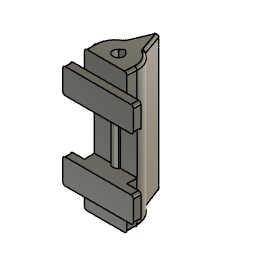
strumballz v18 (Autodesk Fusion 360 design; units mm, degrees)
Autodesk Fusion 360 part; units mm, degrees
note: some values were not read from the file. Chosen so that the rebuilt part matches the saved one: which sketch regions a step uses; which face or edge a step refers to; which pieces of a blend or face edit are solid.
sketch "Sketch1" plane through (0, 0, 0) normal (0, 0, 1) x (1, 0, 0)
  circle A0 centre (0, 0) radius 8.5
  line L0 (0, 8.5) -> (0, 18.5) construction
  line L1 (-8.400646, -4.05702) -> (8.400646, -4.05702)
  line L2 (8.400646, -4.05702) -> (8.497313, -0.213724)
  line L3 (-8.400646, -4.05702) -> (-8.497313, -0.213724)
  line L4 (0, 18.5) -> (-8.400646, -4.05702)
  line L5 (8.400646, -4.05702) -> (0, 18.5)
  dimension "d1" = 17
  dimension "d2" = 10
  constraint coincident A0.centre origin
  constraint coincident A0 L0.start
  constraint vertical L0
  constraint horizontal L1
  constraint tangent A0 L2
  constraint tangent A0 L3
  measures "d1" diameter of A0
  measures "d2" distance of L0.start L0.end
extrude "Extrude1" add sketch "Sketch1" along normal blind 55 contours A0 L5 | A0 L2 L5 | A0 L1 L5 | A0 L1 L4 L5 | A0 L4 L5 | A0 L4 | A0 L1 L4 | A0 L3 L4 picked at (5.724066, 3.776087) picked at (8.210444, -3.009315) picked at (7.842583, -3.934324) picked at (0.204704, 0.121249) picked at (0, 11.818524) picked at (-7.263613, 1.901443) picked at (-7.842583, -3.934324) picked at (-8.210444, -3.009315)
fillet "Fillet1" radius 1 1 edges at (0, 18.5, 27.5)
sketch "Sketch2" plane through (0, 0, 55) normal (0, 0, 1) x (-1, 0, 0)
  arc A0 (-0.937122, -15.983684) -> (0.937122, -15.983684) centre (0, -15.634682) ccw
  line L0 (0.937122, -15.983684) -> (4.121133, -7.434128)
  arc A1 (4.121133, -7.434128) -> (8.497313, 0.213724) centre (0, 0) ccw
  line L1 (8.497313, 0.213724) -> (8.400646, 4.05702)
  line L2 (8.400646, 4.05702) -> (-8.400646, 4.05702)
  line L3 (-8.400646, 4.05702) -> (-8.497313, 0.213724)
  arc A2 (-8.497313, 0.213724) -> (-4.121133, -7.434128) centre (0, 0) ccw
  line L4 (-4.121133, -7.434128) -> (-0.937122, -15.983684)
  line L5 (0, 4.05702) -> (0, -0.94298) construction
  circle A3 centre (0, -0.94298) radius 2.125
  line L6 (0, -3.801151) -> (-1.421105, -2.522881)
  line L7 (0, -3.801151) -> (1.421105, -2.522881)
  dimension "d7" = 5
  dimension "d8" = 4.25
  constraint perpendicular L2 L5
  constraint tangent A3 L6
  constraint tangent A3 L7
  measures "d8" diameter of A3
extrude "Extrude2" cut sketch "Sketch2" against normal up to surface (55 mm away) contours A3 | A3 L6 L7 picked at (0.385258, -0.460245) picked at (0.103405, -3.304782)
fillet "Fillet2" radius 0.5 2 edges at (-4.121133, 7.434128, 27.5) (4.121133, 7.434128, 27.5)
sketch "Sketch3" plane through (0, -4.05702, 0) normal (0, -1, 0) x (1, 0, 0)
  line L0 (-8.400646, 0) -> (8.400646, 0)
  line L1 (8.400646, 0) -> (8.400646, 55)
  line L2 (8.400646, 55) -> (-8.400646, 55)
  line L3 (-8.400646, 55) -> (-8.400646, 0)
  line L4 (0, 55) -> (0, 46.5) construction
  line L5 (0, 0) -> (0, 8.5) construction
  line L6 (14, 55.000001) -> (-14, 55.000001)
  line L7 (-14, 55.000001) -> (-14, 37.999999)
  line L8 (-14, 37.999999) -> (14, 37.999999)
  line L9 (14, 37.999999) -> (14, 55.000001)
  line L10 (14, 55.000001) -> (-14, 37.999999) construction
  line L11 (-14, 55.000001) -> (14, 37.999999) construction
  line L12 (14, 0) -> (-14, 0)
  line L13 (-14, 0) -> (-14, 17)
  line L14 (-14, 17) -> (14, 17)
  line L15 (14, 17) -> (14, 0)
  line L16 (14, 0) -> (-14, 17) construction
  line L17 (-14, 0) -> (14, 17) construction
  line L18 (2, 55.000001) -> (2, 48.000001) construction
  line L19 (14, 48.000001) -> (-14, 48.000001)
  line L20 (13, 0) -> (13, 7) construction
  line L21 (14, 7) -> (-14, 7)
  point P0 (0, 46.5)
  point P1 (0, 8.5)
  dimension "d14" = 8.5
  dimension "d15" = 8.5
  dimension "d36" = 7
  constraint midpoint L2 L4.start
  constraint perpendicular L2 L4
  constraint coincident L5.start origin
  constraint perpendicular L0 L5
  constraint horizontal L6
  constraint perpendicular L6 L7
  constraint parallel L6 L8
  constraint parallel L7 L9
  constraint coincident L10 P0
  constraint coincident L11 P0
  constraint coincident P0 L4.end
  constraint horizontal L12
  constraint perpendicular L12 L13
  constraint parallel L12 L14
  constraint parallel L13 L15
  constraint coincident L16 P1
  constraint coincident L17 P1
  constraint coincident P1 L5.end
  constraint perpendicular L7 L19
  constraint coincident L12 L20.start
  constraint coincident L15 L21.start
  constraint coincident L13 L21.end
  constraint perpendicular L13 L21
  measures "d14" distance of L4.start P0
  measures "d15" distance of L5.start P1
extrude "Extrude3" add sketch "Sketch3" along normal blind 3 contours L3 L13 L14 L21 | L1 L3 L14 L21 | L1 L14 L15 L21 | L3 L7 L8 L19 | L1 L3 L8 L19 | L1 L8 L9 L19 picked at (-10.267098, 10.333333) picked at (2.800215, 10.333333) picked at (10.267098, 13.666667) picked at (-10.267098, 44.666667) picked at (-2.800215, 41.333333) picked at (12.133549, 41.333333)
sketch "Sketch4" plane through (0, -4.05702, 0) normal (0, -1, 0) x (1, 0, 0)
  line L0 (-8.400646, 17) -> (8.400646, 17)
  line L1 (8.400646, 17) -> (8.400646, 37.999999)
  line L2 (8.400646, 37.999999) -> (-8.400646, 37.999999)
  line L3 (-8.400646, 37.999999) -> (-8.400646, 17)
  line L4 (-10, 38.000001) -> (10, 38.000001)
  line L5 (10, 38.000001) -> (10, 17)
  line L6 (10, 17) -> (-10, 17)
  line L7 (-10, 17) -> (-10, 38.000001)
  constraint horizontal L4
  constraint vertical L5
  constraint horizontal L6
  constraint vertical L7
extrude "Extrude4" cut sketch "Sketch4" against normal blind 4 contours L0 L1 L2 L3 L4 L6 | L3 L4 L6 L7 | L1 L4 L5 L6 picked at (2.800215, 24) picked at (-9.466882, 31) picked at (9.466882, 24)
draft "Draft1" angle -2 neutral plane through (0, -0.05702, 0) pull (0, -1, 0) 2 faces at (0.312374, 10.397575, 55) (0.312374, 10.397575, 0)
fillet "Fillet3" radius 1 4 edges at (14, -5.55702, 17) (14, -5.55702, 37.999999) (-14, -5.55702, 37.999999) (-14, -5.55702, 17)
fillet "Fillet4" radius 1 4 edges at (-14, -5.55702, 7) (14, -5.55702, 7) (-14, -5.55702, 48.000001) (14, -5.55702, 48.000001)
fillet "Fillet5" radius 1 11 edges at (8.44898, -2.135372, 55.072578) (-2.497399, 11.794102, 54.58615) (-4.143869, 7.456849, 54.73761) (-7.382537, 4.212854, 54.850893) (-8.498922, -0.135377, 55.002736) (-8.44898, -2.135372, 55.072578) (8.498922, -0.135377, 55.002736) (7.382537, 4.212854, 54.850893) (4.143869, 7.456849, 54.73761) (2.497399, 11.794102, 54.58615) (0, 16.634682, 54.417113)
fillet "Fillet6" radius 1 11 edges at (-2.497399, 11.794102, 0.41385) (-4.143869, 7.456849, 0.26239) (-7.382537, 4.212854, 0.149107) (-8.498922, -0.135377, -0.002736) (-8.44898, -2.135372, -0.072578) (8.44898, -2.135372, -0.072578) (8.498922, -0.135377, -0.002736) (7.382537, 4.212854, 0.149107) (4.143869, 7.456849, 0.26239) (2.497399, 11.794102, 0.41385) (0, 16.634682, 0.582887)
